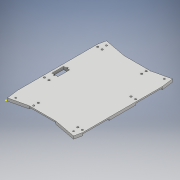
# Autodesk Inventor part: 3枚目
Saved by Autodesk Inventor 2018 (Build 220112000, 112)
## iProperties
Created: 2018-08-16
Part Number: 3枚目
Material: 一般
Document SubType Name: Modeling
Designer: shun2
Density: 1 g/cm^3
Appearance: 既定
Author: shun2
Autodesk Inventor part; units mm, degrees
ref_plane "YZ Plane" through (0, 0, 0) normal (1, 0, 0) x (0, 1, 0)
ref_plane "XZ Plane" through (0, 0, 0) normal (0, 1, 0) x (-1, 0, 0)
ref_plane "XY Plane" through (0, 0, 0) normal (0, 0, 1) x (1, 0, 0)
sketch "スケッチ1" plane through (0, 0, 0) normal (0, 0, 1) x (1, 0, 0)
  circle A0 centre (131.35, 19) radius 1.8
  circle A1 centre (122.35, 19) radius 1.8
  circle A2 centre (4.65, 71) radius 1.8
  circle A3 centre (13.65, 71) radius 1.8
  circle A4 centre (4.65, 175.7239) radius 1.8
  circle A5 centre (13.65, 175.7239) radius 1.8
  circle A6 centre (131.35, 123.7239) radius 1.8
  circle A7 centre (122.35, 123.7239) radius 1.8
  line L0 (0, 179.7239) -> (0, 23)
  line L1 (0, 23) -> (3, 0)
  line L2 (133, 0) -> (136, 15)
  line L3 (136, 15) -> (136, 171.7239)
  line L4 (136, 171.7239) -> (133, 194.7239)
  line L5 (0, 75) -> (18.3, 75)
  line L6 (18.3, 75) -> (18.3, 23)
  line L7 (18.3, 23) -> (0, 23)
  line L8 (0, 23) -> (0, 75)
  line L9 (0, 179.7239) -> (18.3, 179.7239)
  line L10 (18.3, 179.7239) -> (18.3, 127.7239)
  line L11 (18.3, 127.7239) -> (0, 127.7239)
  line L12 (0, 127.7239) -> (0, 179.7239)
  line L13 (46, 186.7239) -> (98, 186.7239)
  line L14 (98, 186.7239) -> (98, 168.4239)
  line L15 (98, 168.4239) -> (46, 168.4239)
  line L16 (46, 168.4239) -> (46, 186.7239)
  line L17 (117.7, 171.7239) -> (136, 171.7239)
  line L18 (136, 171.7239) -> (136, 119.7239)
  line L19 (136, 119.7239) -> (117.7, 119.7239)
  line L20 (117.7, 119.7239) -> (117.7, 171.7239)
  line L21 (117.7, 67) -> (136, 67)
  line L22 (136, 67) -> (136, 15)
  line L23 (136, 15) -> (117.7, 15)
  line L24 (117.7, 15) -> (117.7, 67)
  line L25 (38, 26.3) -> (90, 26.3)
  line L26 (90, 26.3) -> (90, 8)
  line L27 (90, 8) -> (38, 8)
  line L28 (38, 8) -> (38, 26.3)
  circle A8 centre (42, 12.65) radius 1.8
  circle A9 centre (42, 21.65) radius 1.8
  circle A10 centre (94, 182.0739) radius 1.8
  circle A11 centre (94, 173.0739) radius 1.8
  line L29 (3, 194.7239) -> (46, 186.7239)
  line L30 (98, 186.7239) -> (133, 194.7239)
  line L31 (3, 0) -> (38, 8)
  line L32 (38, 8) -> (90, 8)
  line L33 (90, 8) -> (133, 0)
  line L34 (46, 186.7239) -> (98, 186.7239)
  arc A12 (117.7, 160.734) -> (117.655, 160.7883) centre (112.29, 156.292) ccw
  arc A13 (117.655, 151.7957) -> (117.7, 151.8499) centre (112.29, 156.292) ccw
  line L35 (16.4068, 85.862) -> (16.4068, 108.862)
  line L36 (16.4068, 108.862) -> (4.4068, 108.862)
  line L37 (4.4068, 108.862) -> (4.4068, 85.862)
  line L38 (4.4068, 85.862) -> (16.4068, 85.862)
  circle A14 centre (10.4068, 110.362) radius 1.15
  circle A15 centre (10.4068, 84.362) radius 1.15
  line L39 (0, 179.7239) -> (3, 194.7239)
  circle A16 centre (11, 186.7239) radius 1.6
  circle A17 centre (125, 186.7239) radius 1.6
  circle A18 centre (11, 8) radius 1.6
  circle A19 centre (125, 8) radius 1.6
  line L40 (-39.2506, 184.5362) -> (-16.0026, 184.5362)
  line L41 (-16.0026, 184.5362) -> (-13.5186, 184.5362)
  line L42 (-13.5186, 184.5362) -> (-3.2973, 180.8977)
  line L43 (-3.1017, 181.4472) -> (-3.4929, 180.3481)
  line L44 (-3.4929, 180.3481) -> (0, 179.7239)
  line L45 (0, 179.7239) -> (-3.1017, 181.4472)
  line L46 (6.4, 186.7239) -> (15.6, 186.7239)
  line L47 (11, 182.1239) -> (11, 191.3239)
  line L48 (120.4, 186.7239) -> (129.6, 186.7239)
  line L49 (125, 182.1239) -> (125, 191.3239)
  line L50 (6.4, 8) -> (15.6, 8)
  line L51 (11, 3.4) -> (11, 12.6)
  line L52 (120.4, 8) -> (129.6, 8)
  line L53 (125, 3.4) -> (125, 12.6)
  line L54 (3, 194.7239) -> (0, 179.7239)
  line L55 (0, 23) -> (0, 179.7239)
  line L56 (3, 194.7239) -> (46, 186.7239)
  line L57 (46, 186.7239) -> (46, 168.4239)
  line L58 (46, 168.4239) -> (98, 168.4239)
  line L59 (98, 168.4239) -> (98, 186.7239)
  line L60 (133, 194.7239) -> (98, 186.7239)
  line L61 (133, 194.7239) -> (136, 171.7239)
  line L62 (136, 171.7239) -> (136, 15)
  line L63 (136, 15) -> (117.7, 15)
  line L64 (117.7, 15) -> (117.7, 67)
  line L65 (136, 67) -> (117.7, 67)
  line L66 (117.7, 119.7239) -> (136, 119.7239)
  line L67 (117.7, 119.7239) -> (117.7, 171.7239)
  line L68 (117.7, 171.7239) -> (136, 171.7239)
  line L69 (133, 0) -> (136, 15)
  line L70 (90, 8) -> (133, 0)
  line L71 (3, 0) -> (38, 8)
  line L72 (38, 26.3) -> (90, 26.3)
  line L73 (90, 26.3) -> (90, 8)
  line L74 (38, 8) -> (90, 8)
  line L75 (38, 26.3) -> (38, 8)
  line L76 (0, 23) -> (3, 0)
  line L77 (0, 179.7239) -> (18.3, 179.7239)
  line L78 (18.3, 179.7239) -> (18.3, 127.7239)
  line L79 (18.3, 127.7239) -> (0, 127.7239)
  line L80 (0, 127.7239) -> (0, 179.7239)
  line L81 (0, 75) -> (18.3, 75)
  line L82 (18.3, 75) -> (18.3, 23)
  line L83 (18.3, 23) -> (0, 23)
  line L84 (0, 23) -> (0, 75)
  line L85 (0, 127.7239) -> (0, 75)
  circle A20 centre (125, 186.7239) radius 1.6
  circle A21 centre (11, 186.7239) radius 1.6
  circle A22 centre (94, 182.0739) radius 1.8
  circle A23 centre (94, 182.0739) radius 1.8
  circle A24 centre (94, 173.0739) radius 1.8
  circle A25 centre (125, 186.7239) radius 1.6
  circle A26 centre (11, 186.7239) radius 1.6
  circle A27 centre (13.65, 175.7239) radius 1.8
  circle A28 centre (4.65, 175.7239) radius 1.8
  circle A29 centre (122.35, 123.7239) radius 1.8
  circle A30 centre (131.35, 123.7239) radius 1.8
  circle A31 centre (122.35, 19) radius 1.8
  circle A32 centre (131.35, 19) radius 1.8
  circle A33 centre (125, 8) radius 1.6
  circle A34 centre (42, 21.65) radius 1.8
  circle A35 centre (42, 12.65) radius 1.8
  circle A36 centre (4.65, 71) radius 1.8
  circle A37 centre (13.65, 71) radius 1.8
  circle A38 centre (11, 8) radius 1.6
  circle A39 centre (10.4068, 110.362) radius 1.15
  circle A40 centre (10.4068, 84.362) radius 1.15
  line L86 (4.4068, 108.862) -> (16.4068, 108.862)
  line L87 (16.4068, 108.862) -> (16.4068, 85.862)
  line L88 (16.4068, 85.862) -> (4.4068, 85.862)
  line L89 (4.4068, 85.862) -> (4.4068, 108.862)
  line L90 (117.7, 171.7239) -> (136, 171.7239)
  line L91 (136, 171.7239) -> (136, 119.7239)
  line L92 (136, 119.7239) -> (117.7, 119.7239)
  line L93 (117.7, 119.7239) -> (117.7, 171.7239)
  line L94 (117.7, 67) -> (136, 67)
  line L95 (136, 67) -> (136, 15)
  line L96 (136, 15) -> (117.7, 15)
  line L97 (117.7, 15) -> (117.7, 67)
  point P0 (0, 0)
  point P1 (-39.2506, 190.238)
  point P2 (-28.3321, 190.8402)
  constraints: 196 end point, 41 centre point, 21 coincident, 16 concentric, 13 collinear, 12 perpendicular, 10 parallel, 5 horizontal, 4 point on circle, 1 vertical, 4 other
sketch "スケッチ2" plane through (0, 0, 0) normal (0, 0, 1) x (1, 0, 0)
  point P0 (0, 0)
extrude "押し出し1" add sketch "スケッチ1" along normal blind 5.5 contours L39 L29 L16 L15 L14 L30 L4 L17 L20 L19 L3 L21 L24 L23 L2 L33 L26 L25 L28 L31 L1 L7 L6 L5 L0 L11 L10 L9
sketch "スケッチ3" plane through (0, 0, 5.5) normal (0, 0, 1) x (1, 0, 0)
  circle A0 centre (131.35, 19) radius 1.8
  circle A1 centre (122.35, 19) radius 1.8
  circle A2 centre (4.65, 71) radius 1.8
  circle A3 centre (13.65, 71) radius 1.8
  circle A4 centre (4.65, 175.7239) radius 1.8
  circle A5 centre (13.65, 175.7239) radius 1.8
  circle A6 centre (131.35, 123.7239) radius 1.8
  circle A7 centre (122.35, 123.7239) radius 1.8
  line L0 (0, 179.7239) -> (0, 23)
  line L1 (0, 23) -> (3, 0)
  line L2 (133, 0) -> (136, 15)
  line L3 (136, 15) -> (136, 171.7239)
  line L4 (136, 171.7239) -> (133, 194.7239)
  line L5 (0, 75) -> (18.3, 75)
  line L6 (18.3, 75) -> (18.3, 23)
  line L7 (18.3, 23) -> (0, 23)
  line L8 (0, 23) -> (0, 75)
  line L9 (0, 179.7239) -> (18.3, 179.7239)
  line L10 (18.3, 179.7239) -> (18.3, 127.7239)
  line L11 (18.3, 127.7239) -> (0, 127.7239)
  line L12 (0, 127.7239) -> (0, 179.7239)
  line L13 (46, 186.7239) -> (98, 186.7239)
  line L14 (98, 186.7239) -> (98, 168.4239)
  line L15 (98, 168.4239) -> (46, 168.4239)
  line L16 (46, 168.4239) -> (46, 186.7239)
  line L17 (117.7, 171.7239) -> (136, 171.7239)
  line L18 (136, 171.7239) -> (136, 119.7239)
  line L19 (136, 119.7239) -> (117.7, 119.7239)
  line L20 (117.7, 119.7239) -> (117.7, 171.7239)
  line L21 (117.7, 67) -> (136, 67)
  line L22 (136, 67) -> (136, 15)
  line L23 (136, 15) -> (117.7, 15)
  line L24 (117.7, 15) -> (117.7, 67)
  line L25 (38, 26.3) -> (90, 26.3)
  line L26 (90, 26.3) -> (90, 8)
  line L27 (90, 8) -> (38, 8)
  line L28 (38, 8) -> (38, 26.3)
  circle A8 centre (42, 12.65) radius 1.8
  circle A9 centre (42, 21.65) radius 1.8
  circle A10 centre (94, 182.0739) radius 1.8
  circle A11 centre (94, 173.0739) radius 1.8
  line L29 (3, 194.7239) -> (46, 186.7239)
  line L30 (98, 186.7239) -> (133, 194.7239)
  line L31 (3, 0) -> (38, 8)
  line L32 (38, 8) -> (90, 8)
  line L33 (90, 8) -> (133, 0)
  line L34 (46, 186.7239) -> (98, 186.7239)
  circle A12 centre (23.71, 156.292) radius 1.59
  circle A13 centre (112.29, 156.292) radius 1.59
  circle A14 centre (112.29, 38.432) radius 1.59
  circle A15 centre (23.71, 38.432) radius 1.59
  arc A16 (105.29, 161.292) -> (112.29, 149.292) centre (112.8589, 157.6655) ccw
  arc A17 (23.71, 149.292) -> (30.71, 161.292) centre (23.1411, 157.6655) ccw
  arc A18 (117.7, 160.734) -> (117.655, 160.7883) centre (112.29, 156.292) ccw
  arc A19 (117.655, 151.7957) -> (117.7, 151.8499) centre (112.29, 156.292) ccw
  line L35 (30.71, 161.292) -> (105.29, 161.292)
  arc A20 (30.71, 33.432) -> (23.71, 45.432) centre (23.1411, 37.0584) ccw
  arc A21 (112.29, 45.432) -> (105.29, 33.432) centre (112.8589, 37.0584) ccw
  line L36 (23.71, 45.432) -> (23.71, 149.292)
  line L37 (112.29, 149.292) -> (112.29, 45.432)
  line L38 (16.4068, 85.862) -> (16.4068, 108.862)
  line L39 (16.4068, 108.862) -> (4.4068, 108.862)
  line L40 (4.4068, 108.862) -> (4.4068, 85.862)
  line L41 (4.4068, 85.862) -> (16.4068, 85.862)
  circle A22 centre (10.4068, 110.362) radius 1.15
  circle A23 centre (10.4068, 84.362) radius 1.15
  line L42 (0, 179.7239) -> (3, 194.7239)
  line L43 (30.71, 33.432) -> (105.29, 33.432)
  circle A24 centre (11, 186.7239) radius 1.6
  circle A25 centre (125, 186.7239) radius 1.6
  circle A26 centre (11, 8) radius 1.6
  circle A27 centre (125, 8) radius 1.6
  line L44 (-39.2506, 184.5362) -> (-16.0026, 184.5362)
  line L45 (-16.0026, 184.5362) -> (-13.5186, 184.5362)
  line L46 (-13.5186, 184.5362) -> (-3.2973, 180.8977)
  line L47 (-3.1017, 181.4472) -> (-3.4929, 180.3481)
  line L48 (-3.4929, 180.3481) -> (0, 179.7239)
  line L49 (0, 179.7239) -> (-3.1017, 181.4472)
  line L50 (6.4, 186.7239) -> (15.6, 186.7239)
  line L51 (11, 182.1239) -> (11, 191.3239)
  line L52 (120.4, 186.7239) -> (129.6, 186.7239)
  line L53 (125, 182.1239) -> (125, 191.3239)
  line L54 (6.4, 8) -> (15.6, 8)
  line L55 (11, 3.4) -> (11, 12.6)
  line L56 (120.4, 8) -> (129.6, 8)
  line L57 (125, 3.4) -> (125, 12.6)
  line L58 (0, 179.7239) -> (18.3, 179.7239) projected
  line L59 (18.3, 179.7239) -> (18.3, 127.7239) projected
  line L60 (0, 179.7239) -> (18.3, 179.7239)
  line L61 (18.3, 179.7239) -> (18.3, 127.7239)
  line L62 (18.3, 127.7239) -> (0, 127.7239)
  line L63 (0, 127.7239) -> (0, 179.7239)
  line L64 (46, 168.4239) -> (46, 186.7239) projected
  line L65 (98, 168.4239) -> (46, 168.4239) projected
  line L66 (46, 186.7239) -> (98, 186.7239)
  line L67 (98, 186.7239) -> (98, 168.4239)
  line L68 (98, 168.4239) -> (46, 168.4239)
  line L69 (46, 168.4239) -> (46, 186.7239)
  line L70 (136, 119.7239) -> (117.7, 119.7239)
  line L71 (117.7, 119.7239) -> (117.7, 171.7239)
  line L72 (117.7, 171.7239) -> (136, 171.7239)
  line L73 (136, 171.7239) -> (136, 119.7239)
  line L74 (117.7, 67) -> (136, 67)
  line L75 (136, 67) -> (136, 15)
  line L76 (136, 15) -> (117.7, 15)
  line L77 (117.7, 15) -> (117.7, 67)
  line L78 (38, 26.3) -> (90, 26.3) projected
  line L79 (90, 8) -> (38, 8)
  line L80 (38, 8) -> (38, 26.3)
  line L81 (38, 26.3) -> (90, 26.3)
  line L82 (90, 26.3) -> (90, 8)
  line L83 (18.3, 23) -> (0, 23)
  line L84 (0, 23) -> (0, 75)
  line L85 (0, 75) -> (18.3, 75)
  line L86 (18.3, 75) -> (18.3, 23)
  circle A28 centre (4.65, 175.7239) radius 1.8
  circle A29 centre (13.65, 175.7239) radius 1.8
  circle A30 centre (94, 182.0739) radius 1.8
  circle A31 centre (94, 173.0739) radius 1.8
  circle A32 centre (122.35, 123.7239) radius 1.8
  circle A33 centre (131.35, 123.7239) radius 1.8
  circle A34 centre (122.35, 19) radius 1.8
  circle A35 centre (131.35, 19) radius 1.8
  circle A36 centre (42, 21.65) radius 1.8
  circle A37 centre (42, 12.65) radius 1.8
  circle A38 centre (4.65, 71) radius 1.8
  circle A39 centre (13.65, 71) radius 1.8
  point P0 (0, 0)
  point P1 (-39.2506, 190.238)
  point P2 (-28.3321, 190.8402)
  constraints: 164 end point, 40 centre point, 12 coincident, 12 concentric, 12 parallel, 12 point on circle, 6 horizontal, 6 perpendicular, 2 other
extrude "押し出し2" add sketch "スケッチ3" against normal blind 2.5 contours L9 L10 L11 L0 | L5 L6 L7 L0 | L13 L14 L15 L16 | L28 L25 L26 L27 | L3 L19 L20 L17 | L3 L23 L24 L21
